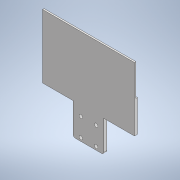
# Autodesk Inventor part: lead_1
Saved by Autodesk Inventor 2022 (Build 260153000, 153)
## iProperties
Created: 2022-12-25
Part Number: lead_1
Material: Lead
Document SubType Name: Modeling
Designer: Kamil
Mass: 173.129 g
Surface Area: 141.135 cm^2
Volume: 15.2671 cm^3
Density: 11.34 g/cm^3
Appearance: Lead
Author: Kamil
Autodesk Inventor part; units mm, degrees
ref_plane "YZ Plane" through (0, 0, 0) normal (1, 0, 0) x (0, 1, 0)
ref_plane "XZ Plane" through (0, 0, 0) normal (0, 1, 0) x (-1, 0, 0)
ref_plane "XY Plane" through (0, 0, 0) normal (0, 0, 1) x (1, 0, 0)
sketch "Sketch1" plane through (0, 0, 0) normal (0, 0, 1) x (1, 0, 0)
  line L0 (-15, -28.975) -> (-15, -0.175) projected
  arc A0 (-15, -28.975) -> (-13, -30.975) centre (-13, -28.975) ccw projected
  line L1 (13, -30.975) -> (-13, -30.975) projected
  arc A1 (13, -30.975) -> (15, -28.975) centre (13, -28.975) ccw projected
  line L2 (15, -0.175) -> (15, -28.975) projected
  line L3 (45, -0.175) -> (15, -0.175) projected
  line L4 (45, 62.125) -> (45, -0.175) projected
  line L5 (-15, -0.175) -> (-45, -0.175) projected
  circle A2 centre (7.5, -27.775) radius 1.75 projected
  circle A3 centre (7.5, -9.775) radius 1.75 projected
  circle A4 centre (-7.5, -9.775) radius 1.75 projected
  circle A5 centre (-7.5, -27.775) radius 1.75 projected
  line L6 (-45, 62.125) -> (45, 62.125) projected
  line L7 (-45, -0.175) -> (-45, 62.125) projected
  point P0 (0, 0)
  point P1 (-45, 30.975)
extrude "Extrusion1" add sketch "Sketch1" along normal blind 1.5
sketch "Sketch2" plane through (0, 0, 1.5) normal (0, 0, 1) x (1, 0, 0)
  line L0 (-45, 30.975) -> (45, 30.975) projected
  line L1 (45, 62.125) -> (45, 30.975) projected
  line L2 (-45, 62.125) -> (45, 62.125) projected
  line L3 (-45, 30.975) -> (-45, 62.125) projected
  line L4 (15, -28.975) -> (15, -0.175) projected
  line L5 (15, -0.175) -> (45, -0.175) projected
  line L6 (45, -0.175) -> (45, 62.125) projected
  line L7 (-45, -0.175) -> (-15, -0.175) projected
  line L8 (-15, -0.175) -> (-15, -28.975) projected
  arc A0 (-15, -28.975) -> (-13, -30.975) centre (-13, -28.975) ccw projected
  line L9 (-13, -30.975) -> (13, -30.975) projected
  arc A1 (13, -30.975) -> (15, -28.975) centre (13, -28.975) ccw projected
  circle A2 centre (7.5, -27.775) radius 1.75 projected
  circle A3 centre (7.5, -9.775) radius 1.75 projected
  circle A4 centre (-7.5, -9.775) radius 1.75 projected
  circle A5 centre (-7.5, -27.775) radius 1.75 projected
  line L10 (45, 62.125) -> (-45, 62.125) projected
  line L11 (-45, 62.125) -> (-45, -0.175) projected
  point P0 (0, 0)
extrude "Extrusion2" add sketch "Sketch2" along normal blind 1.5
sketch "Sketch3" plane through (0, 0, 3) normal (0, 0, 1) x (1, 0, 0)
  line L0 (45, 62.125) -> (-45, 62.125) projected
  line L1 (-45, 62.125) -> (-45, -0.175) projected
  line L2 (-45, -0.175) -> (-15, -0.175) projected
  line L3 (-15, -0.175) -> (-15, -28.975) projected
  arc A0 (-15, -28.975) -> (-13, -30.975) centre (-13, -28.975) ccw projected
  line L4 (-13, -30.975) -> (13, -30.975) projected
  arc A1 (13, -30.975) -> (15, -28.975) centre (13, -28.975) ccw projected
  line L5 (15, -28.975) -> (15, -0.175) projected
  line L6 (15, -0.175) -> (45, -0.175) projected
  line L7 (45, -0.175) -> (45, 62.125) projected
  circle A2 centre (7.5, -27.775) radius 1.75 projected
  circle A3 centre (7.5, -9.775) radius 1.75 projected
  circle A4 centre (-7.5, -9.775) radius 1.75 projected
  circle A5 centre (-7.5, -27.775) radius 1.75 projected
  circle A6 centre (0, -18.775) radius 2.6186 projected
  line L8 (-13, -30.975) -> (13, -30.975) projected
  line L9 (0, -13.8344) -> (4.5, -13.8344)
  line L10 (4.5, -13.8344) -> (4.5, -30.975)
  line L11 (4.5, -30.975) -> (0, -30.975)
  line L12 (0, -30.975) -> (0, -13.8344)
  line L13 (0, -13.8344) -> (-4.5, -13.8344)
  line L14 (-4.5, -13.8344) -> (-4.5, -30.975)
  point P0 (0, 0)
  dimension "d4" = 4.5
  constraints: 12 end point, 2 parallel, 2 symmetric about line, 1 horizontal, 1 perpendicular, 1 point on line
  measures "d4" distance of L10.end L11.end
extrude "Extrusion3" cut sketch "Sketch3" against normal through all contours L4 L12 A6 L9 L10 | L14 L13 L12 A6 L4 | L12 A6 | A6 L12
sketch "Sketch4" plane through (0, 0, 1.5) normal (0, 0, -1) x (-1, 0, 0)
  circle A0 centre (7.5, -27.775) radius 1.75 projected
  circle A1 centre (7.5, -9.775) radius 1.75 projected
  circle A2 centre (-7.5, -9.775) radius 1.75 projected
  circle A3 centre (-7.5, -27.775) radius 1.75 projected
  line L0 (4.5, -30.975) -> (4.5, -13.8344) projected
  line L1 (4.5, -13.8344) -> (-4.5, -13.8344) projected
  line L2 (-4.5, -13.8344) -> (-4.5, -30.975) projected
  line L3 (-4.5, -30.975) -> (-13, -30.975) projected
  arc A4 (-15, -28.975) -> (-13, -30.975) centre (-13, -28.975) ccw projected
  line L4 (-15, -28.975) -> (-15, -0.175) projected
  line L5 (-15, -0.175) -> (-45, -0.175) projected
  line L6 (-45, -0.175) -> (-45, 62.125) projected
  line L7 (-45, 62.125) -> (45, 62.125) projected
  line L8 (45, 62.125) -> (45, -0.175) projected
  line L9 (45, -0.175) -> (15, -0.175) projected
  line L10 (15, -0.175) -> (15, -28.975) projected
  arc A5 (13, -30.975) -> (15, -28.975) centre (13, -28.975) ccw projected
  line L11 (13, -30.975) -> (4.5, -30.975) projected
  line L12 (-45, 30.975) -> (45, 30.975) projected
  point P0 (0, 0)
extrude "Extrusion4" [suppressed]
body "Solid1"
